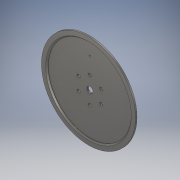
# Autodesk Inventor part: FrontDisk
Saved by Autodesk Inventor 2019.4 (Build 234330000, 330)
## iProperties
Created: 2020-09-30
Part Number: FrontDisk
Material: Steel, Alloy
Document SubType Name: Modeling
Designer: Federico
Density: 7.73 g/cm^3
Appearance: Semi-Polished
Author: Federico
Autodesk Inventor part; units mm, degrees
ref_plane "YZ Plane" through (0, 0, 0) normal (1, 0, 0) x (0, 1, 0)
ref_plane "XZ Plane" through (0, 0, 0) normal (0, 1, 0) x (-1, 0, 0)
sketch "Sketch1" plane through (0, 0, 0) normal (0, 0, 1) x (1, 0, 0)
  circle A0 centre (0, 0) radius 155
  circle A1 centre (0, 0) radius 10
  circle A2 centre (0, 0) radius 137
  dimension "d0" = 310
  dimension "d1" = 20
  dimension "d2" = 274
  constraints: 3 centre point, 3 coincident
  measures "d0" diameter of A0
  measures "d1" diameter of A1
  measures "d2" diameter of A2
extrude "Extrusion1" add sketch "Sketch1" along normal blind 5 contours A0
extrude "Extrusion2" add sketch "Sketch1" against normal blind 5 contours A2
sketch "Sketch2" plane through (0, 0, 0) normal (0, 0, 1) x (1, 0, 0)
  circle A0 centre (0, 43) radius 5
  circle A1 centre (-37.2391, 21.5) radius 5
  circle A2 centre (-37.2391, -21.5) radius 5
  circle A3 centre (0, -43) radius 5
  circle A4 centre (37.2391, -21.5) radius 5
  circle A5 centre (37.2391, 21.5) radius 5
  point P0 (0, 0)
  point P1 (0, 0)
  point P2 (0, 0)
  point P3 (0, 0)
  point P4 (0, 0)
  point P5 (0, 0)
  point P6 (0, 0)
  point P7 (0, 0)
  point P8 (0, 0)
  point P9 (0, 0)
  point P10 (0, 0)
  point P11 (0, 0)
  dimension "d10" = 10
  dimension "d11" = 43
  dimension "d9" = 360
  constraints: 8 coincident, 6 centre point, 23 other
  measures "d10" diameter of A0
  measures "d11" distance of point (0, 0) A0.centre
extrude "Extrusion3" cut sketch "Sketch2" against normal blind 5
chamfer "Chamfer1" distance 4 angle 45 1 edges at (-137, 0, 5)
chamfer "Chamfer2" distance 4 angle 45 1 edges at (-137, 0, -5)
ref_plane "Work Plane1" through (0, 0, 0) normal (0, 0, 1) x (1, 0, 0)
sketch "Sketch3" plane through (0, 0, 0) normal (0, 0, 1) x (1, 0, 0)
  circle A0 centre (0, 97) radius 2.5
  line L0 (0, 97) -> (0, 137)
  circle A1 centre (0, 0) radius 137 projected
  dimension "d23" = 5
  dimension "d26" = 40
  constraints: 2 end point, 1 centre point, 1 vertical, 1 vertical alignment, 1 other
  measures "d23" diameter of A0
  measures "d26" distance of L0.start L0.end
extrude "Extrusion4" cut sketch "Sketch3" against normal blind 5 contours A0
body "Solid1"
